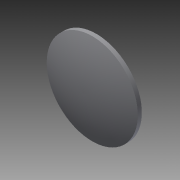
# Autodesk Inventor part: MellesGriot01MCG023
Saved by Autodesk Inventor 2014 (Build 180170000, 170)
## iProperties
Created: 2014-05-16
Part Number: MellesGriot01MCG023
Material: Generic
Document SubType Name: Modeling
Designer: ijs09
Density: 1 g/cm^3
Appearance: Default
Author: ijs09
Autodesk Inventor part; units mm, degrees
ref_plane "YZ Plane" through (0, 0, 0) normal (1, 0, 0) x (0, 1, 0)
ref_plane "XZ Plane" through (0, 0, 0) normal (0, 1, 0) x (-1, 0, 0)
ref_plane "XY Plane" through (0, 0, 0) normal (0, 0, 1) x (1, 0, 0)
sketch "Sketch1" plane through (0, 0, 0) normal (0, 0, 1) x (1, 0, 0)
  line L0 (0, 0) -> (0, 4)
  line L1 (-45, 8.4375) -> (-45, 12.4375)
  arc A0 (-45, 8.4375) -> (0, 0) centre (-0.9646, 119.0743) ccw
  arc A1 (-45, 12.4375) -> (0, 4) centre (-2.3036, 115.9331) ccw
  dimension "d0" = 45
  dimension "d1" = 4
  dimension "d2" = 4
  constraints: 4 end point, 4 point on circle, 2 centre point, 1 parallel, 1 vertical
  measures "d0" distance between parallel lines of L1 L0
  measures "d1" distance of L1.start L1.end
  measures "d2" distance of L0.start L0.end
revolve "Revolution1" add sketch "Sketch1" angle 360 about axis through (0, 0, 0) along (0, 1, 0)
body "Solid1"
